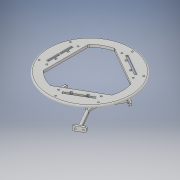
# Autodesk Inventor part: Stewart-Platform-Base-Außenanordnung
Saved by Autodesk Inventor 2018.2 (Build 222227000, 227)
## iProperties
Created: 2018-02-17
Part Number: Stewart-Platform-Base-Außenanordnung
Material: Generisch
Document SubType Name: Modeling
Designer: JochenAlt
Density: 1 g/cm^3
Appearance: Vorgabe
Author: JochenAlt
Autodesk Inventor part; units mm, degrees
ref_plane "YZ Plane" through (0, 0, 0) normal (1, 0, 0) x (0, 1, 0)
ref_plane "XZ Plane" through (0, 0, 0) normal (0, 1, 0) x (-1, 0, 0)
sketch "Skizze1" plane through (0, 0, 0) normal (0, 0, 1) x (1, 0, 0)
  line L0 (0, 96.3661) -> (0, -97.9027) construction
  line L1 (-96.2838, 0) -> (97.409, 0) construction
  line L2 (-57.6011, 28.85) -> (-45.1011, 28.85) construction
  line L3 (-41.8011, 25.55) -> (-41.8011, -25.55) construction
  line L4 (-45.1011, -28.85) -> (-57.6011, -28.85) construction
  line L5 (-60.9011, -25.55) -> (-60.9011, 25.55) construction
  arc A0 (-57.6011, 28.85) -> (-60.9011, 25.55) centre (-57.6011, 25.55) ccw construction
  arc A1 (-41.8011, 25.55) -> (-45.1011, 28.85) centre (-45.1011, 25.55) ccw construction
  arc A2 (-45.1011, -28.85) -> (-41.8011, -25.55) centre (-45.1011, -25.55) ccw construction
  arc A3 (-60.9011, -25.55) -> (-57.6011, -28.85) centre (-57.6011, -25.55) ccw construction
  circle A4 centre (-57.6011, 25.55) radius 1.3
  circle A5 centre (-45.1011, 25.55) radius 1.3
  circle A6 centre (-57.6011, -25.55) radius 1.3
  circle A7 centre (-45.1011, -25.55) radius 1.3
  line L6 (-47.8011, 20.25) -> (-47.8011, -20.25)
  line L7 (-50.9011, 20.25) -> (-50.9011, -20.25)
  line L8 (-50.9011, 20.25) -> (-47.8011, 20.25)
  line L9 (-50.9011, -20.25) -> (-47.8011, -20.25)
  line L10 (-50.9011, 0.8) -> (-47.8011, 0.8)
  line L11 (-50.9011, -0.8) -> (-47.8011, -0.8)
  line L12 (-47.8011, 11.55) -> (-44.7851, 11.55)
  line L13 (-44.7851, 11.55) -> (-44.7851, 8.75)
  line L14 (-44.7851, 8.75) -> (-47.8011, 8.75)
  line L15 (-47.8011, -8.75) -> (-44.7851, -8.75)
  line L16 (-44.7851, -8.75) -> (-44.7851, -11.55)
  line L17 (-44.7851, -11.55) -> (-47.8011, -11.55)
  line L18 (-45.1011, 29.15) -> (-57.6011, 29.15)
  arc A8 (-57.6011, 29.15) -> (-61.2011, 25.55) centre (-57.6011, 25.55) ccw
  line L19 (-61.2011, 25.55) -> (-61.2011, -25.55)
  arc A9 (-61.2011, -25.55) -> (-57.6011, -29.15) centre (-57.6011, -25.55) ccw
  line L20 (-57.6011, -29.15) -> (-45.1011, -29.15)
  arc A10 (-45.1011, -29.15) -> (-41.5011, -25.55) centre (-45.1011, -25.55) ccw
  line L21 (-41.5011, -25.55) -> (-41.5011, 25.55)
  arc A11 (-41.5011, 25.55) -> (-45.1011, 29.15) centre (-45.1011, 25.55) ccw
  line L22 (-63.3321, -28.8235) -> (-60.7271, -27.3356) construction
  line L23 (-39.5011, 0) -> (-41.5011, 0) construction
  circle A12 centre (0, 0) radius 39.5011 construction
  circle A13 centre (0, 0) radius 68.6134
  line L24 (-62.7201, 27.8206) -> (-60.8919, 27.0097) construction
  line L25 (-44.7851, -10.15) -> (-5.8601, -10.15) construction
  line L26 (6.3855, -31.3601) -> (-5.8601, -10.15) construction
  line L27 (-40.5011, -10.15) -> (-40.5011, -70.15) construction
  line L28 (11.4604, -40.15) -> (-40.5011, -70.15) construction
  line L29 (-41.5011, -19.95) -> (-47.8011, -19.95)
  line L30 (-41.5011, 19.95) -> (-47.8011, 19.95)
  arc A14 (47.7952, -24.4837) -> (42.8775, -23.166) centre (44.6775, -26.2837) ccw
  circle A15 centre (44.6775, -26.2837) radius 1.3
  line L31 (42.8775, -23.166) -> (-1.3764, -48.716)
  line L32 (38.0278, -25.966) -> (41.1778, -31.422)
  line L33 (32.3952, -33.0101) -> (33.9032, -35.622)
  line L34 (29.9703, -34.4101) -> (32.3952, -33.0101)
  line L35 (31.4783, -37.022) -> (29.9703, -34.4101)
  line L36 (6.3635, -51.522) -> (41.4376, -31.272)
  line L37 (42.9876, -33.9567) -> (41.4376, -31.272)
  line L38 (7.9135, -54.2067) -> (42.9876, -33.9567)
  line L39 (26.1434, -43.6817) -> (24.5934, -40.997)
  line L40 (24.7577, -44.4817) -> (23.2077, -41.797)
  line L41 (12.39, -44.5601) -> (14.8148, -43.1601)
  line L42 (14.8148, -43.1601) -> (16.3228, -45.772)
  line L43 (13.898, -47.172) -> (12.39, -44.5601)
  line L44 (3.4734, -45.916) -> (6.6234, -51.372)
  line L45 (7.9135, -54.2067) -> (6.3635, -51.522)
  arc A16 (-1.3764, -48.716) -> (-2.6941, -53.6337) centre (0.4236, -51.8337) ccw
  circle A17 centre (0.4236, -51.8337) radius 1.3
  line L46 (-2.6941, -53.6337) -> (3.5559, -64.459)
  circle A18 centre (50.9275, -37.109) radius 1.3
  arc A19 (52.7275, -40.2267) -> (54.0452, -35.309) centre (50.9275, -37.109) ccw
  line L47 (8.4736, -65.7767) -> (52.7275, -40.2267)
  circle A20 centre (6.6736, -62.659) radius 1.3
  arc A21 (3.5559, -64.459) -> (8.4736, -65.7767) centre (6.6736, -62.659) ccw
  line L48 (54.0452, -35.309) -> (47.7952, -24.4837)
  arc A22 (-2.6941, 53.6337) -> (-1.3764, 48.716) centre (0.4236, 51.8337) ccw
  circle A23 centre (0.4236, 51.8337) radius 1.3
  line L49 (-1.3764, 48.716) -> (42.8775, 23.166)
  line L50 (3.4734, 45.916) -> (6.6234, 51.372)
  line L51 (12.39, 44.5601) -> (13.898, 47.172)
  line L52 (14.8148, 43.1601) -> (12.39, 44.5601)
  line L53 (16.3228, 45.772) -> (14.8148, 43.1601)
  line L54 (41.4376, 31.272) -> (6.3635, 51.522)
  line L55 (7.9135, 54.2067) -> (6.3635, 51.522)
  line L56 (42.9876, 33.9567) -> (7.9135, 54.2067)
  line L57 (24.7577, 44.4817) -> (23.2077, 41.797)
  line L58 (26.1434, 43.6817) -> (24.5934, 40.997)
  line L59 (32.3952, 33.0101) -> (29.9703, 34.4101)
  line L60 (29.9703, 34.4101) -> (31.4783, 37.022)
  line L61 (33.9032, 35.622) -> (32.3952, 33.0101)
  line L62 (38.0278, 25.966) -> (41.1778, 31.422)
  line L63 (42.9876, 33.9567) -> (41.4376, 31.272)
  arc A24 (42.8775, 23.166) -> (47.7952, 24.4837) centre (44.6775, 26.2837) ccw
  circle A25 centre (44.6775, 26.2837) radius 1.3
  line L64 (47.7952, 24.4837) -> (54.0452, 35.309)
  circle A26 centre (6.6736, 62.659) radius 1.3
  arc A27 (8.4736, 65.7767) -> (3.5559, 64.459) centre (6.6736, 62.659) ccw
  line L65 (52.7275, 40.2267) -> (8.4736, 65.7767)
  circle A28 centre (50.9275, 37.109) radius 1.3
  arc A29 (54.0452, 35.309) -> (52.7275, 40.2267) centre (50.9275, 37.109) ccw
  line L66 (3.5559, 64.459) -> (-2.6941, 53.6337)
  line L67 (-39.5011, 36.0231) -> (-39.5011, -36.0231)
  line L68 (50.9475, -16.1974) -> (-11.4464, -52.2205)
  arc A30 (-53.749, 29.15) -> (-53.9107, 28.85) centre (0, 0) ccw
  arc A31 (-38.9435, -37.4086) -> (-12.9251, -52.4304) centre (0, 0) ccw
  line L69 (68.3365, 6.1578) -> (69.7386, 5.3484)
  arc A32 (51.8686, -15.0217) -> (51.8686, 15.0217) centre (0, 0) ccw
  arc A33 (-12.9251, 52.4304) -> (-38.9435, 37.4086) centre (0, 0) ccw
  line L70 (-30.7811, 63.3834) -> (-28.8354, 62.2601)
  line L71 (-11.4464, 52.2205) -> (50.9475, 16.1974)
  arc A34 (-39.5011, -36.0231) -> (-38.9435, -37.4086) centre (-37.5011, -36.0231) ccw
  arc A35 (-12.9251, -52.4304) -> (-11.4464, -52.2205) centre (-12.4464, -50.4885) ccw
  arc A36 (50.9475, -16.1974) -> (51.8686, -15.0217) centre (49.9475, -14.4654) ccw
  arc A37 (51.8686, 15.0217) -> (50.9475, 16.1974) centre (49.9475, 14.4654) ccw
  arc A38 (-11.4464, 52.2205) -> (-12.9251, 52.4304) centre (-12.4464, 50.4885) ccw
  arc A39 (-38.9435, 37.4086) -> (-39.5011, 36.0231) centre (-37.5011, 36.0231) ccw
  point P0 (0, 2)
  point P1 (-41.5011, -21.4)
  point P2 (-41.5011, 21.4)
  point P3 (20.7506, -35.941)
  point P4 (39.2835, -25.241)
  point P5 (2.2176, -46.641)
  point P6 (31.1827, -33.7101)
  point P7 (54.0368, -38.9234)
  point P8 (7.0549, -66.2388)
  point P9 (20.7506, 35.941)
  point P10 (2.2176, 46.641)
  point P11 (39.2835, 25.241)
  point P12 (13.6024, 43.8601)
  point P13 (6.6903, 66.259)
  point P14 (53.837, 39.2291)
  point P15 (-39.5011, 36.8193)
  point P16 (-39.5011, -36.8193)
  point P17 (51.637, -15.7993)
  point P18 (-12.1359, -52.6186)
  point P19 (51.637, 15.7993)
  point P20 (-12.1359, 52.6186)
  dimension "d1" = 57.7
  dimension "d2" = 19.1
  dimension "d3" = 3.3
  dimension "d5" = 2.6
  dimension "d6" = 6
  dimension "d7" = 3.1
  dimension "d9" = 1.6
  dimension "d10" = 2.984
  dimension "d11" = 2.8
  dimension "d12" = 17.5
  dimension "d21" = 0.3
  dimension "d22" = 3
  dimension "d34" = 2
  dimension "d35" = 2
  dimension "d40" = 1
  dimension "d42" = 60
  dimension "d43" = 137.2269
  dimension "d105" = 360
  dimension "d107" = 40.5
  dimension "d108" = 0.3
  dimension "d109" = 1
  dimension "d110" = 54
  dimension "d111" = 2
  constraints: 134 end point, 67 point on circle, 39 centre point, 33 point on line, 20 tangent, 14 coincident, 13 equal radius, 11 horizontal, 8 parallel, 6 perpendicular, 4 vertical, 3 line through centre, 2 midpoint, 1 collinear, 1 horizontal alignment, 258 other
  measures "d1" distance between parallel lines of L4 L2
  measures "d2" distance between parallel lines of L3 L5
  measures "d3" radius of A0
  measures "d5" diameter of A4
  measures "d9" distance between parallel lines of L11 L10
  measures "d10" distance between parallel lines of L3 L13
  measures "d11" distance between parallel lines of L14 L12
  measures "d12" distance between parallel lines of L15 L14
  measures "d21" distance between parallel lines of L19 L5
  measures "d22" distance of L22.end L22.start
  measures "d34" distance of L23.start L23.end
  measures "d35" distance of L24.start L24.end
  measures "d40" distance between parallel lines of L21 L27
  measures "d42" distance from line of L25 L27.end
  measures "d43" diameter of A13
  measures "d107" distance between parallel lines of L8 L9
  measures "d108" distance between parallel lines of L29 L9
  measures "d109" distance between parallel lines of L28 L31
  measures "d110" radius of A33
  measures "d111" radius of A34
extrude "Extrusion5" add sketch "Skizze1" along normal blind 4 contours L8 L7 L9 L6 L29 L21 A10 L20 A9 L19 A8 L18 A11 L30 | L30 L21 L29 L6 L17 L16 L15 L14 L13 L12 | L10 L6 L11 L7 | A13 | L48 A19 L47 A21 L46 A16 L31 L44 L36 L45 L38 L37 L32 A14 | L32 L36 L33 L34 L35 L42 L41 L43 L44 L31 | L66 A27 L65 A29 L64 A24 L49 L62 L54 L63 L56 L55 L50 A22 | L50 L54 L51 L52 L53 L60 L59 L61 L62 L49
extrude "Extrusion4" cut sketch "Skizze1" along normal blind 2 contours L8 L7 L9 L6 L29 L21 A10 L20 A9 L19 A8 L18 A11 L30 | L48 A19 L47 A21 L46 A16 L31 L44 L36 L45 L38 L37 L32 A14 | L66 A27 L65 A29 L64 A24 L49 L62 L54 L63 L56 L55 L50 A22
ref_plane "Arbeitsebene2" through (0, 0, -41.8) normal (0, 0, 1) x (1, 0, 0)
sketch "Skizze6" plane through (0, 0, -41.8) normal (0, 0, 1) x (1, 0, 0)
  line L0 (-47.8011, -0.8) -> (-47.8011, -8.75) construction
  line L1 (-47.8011, -8.75) -> (-44.7851, -8.75) construction
  line L2 (-44.7851, -8.75) -> (-44.7851, -11.55) construction
  line L3 (-44.7851, -11.55) -> (-47.8011, -11.55) construction
  line L4 (-47.8011, -11.55) -> (-47.8011, -20.25) construction
  line L5 (-47.8011, -20.25) -> (-50.9011, -20.25) construction
  line L6 (-50.9011, -20.25) -> (-50.9011, -0.8) construction
  line L7 (-47.8011, 20.25) -> (-47.8011, 11.55) construction
  line L8 (-47.8011, 11.55) -> (-44.7851, 11.55) construction
  line L9 (-44.7851, 11.55) -> (-44.7851, 8.75) construction
  line L10 (-44.7851, 8.75) -> (-47.8011, 8.75) construction
  line L11 (-50.9011, 20.25) -> (-47.8011, 20.25) construction
  circle A0 centre (-45.1011, -25.55) radius 1.3 construction
  circle A1 centre (-57.6011, -25.55) radius 1.3 construction
  circle A2 centre (-45.1011, 25.55) radius 1.3 construction
  circle A3 centre (-57.6011, 25.55) radius 1.3 construction
  circle A4 centre (0, 0) radius 68.6134 construction
  line L12 (-47.8011, -8.75) -> (-47.8011, 8.75)
  line L13 (-47.8011, -8.75) -> (-44.7851, -8.75)
  line L14 (-47.8011, 8.75) -> (-47.8011, -8.75) projected
  line L15 (-94.5835, 0) -> (94.5835, 0) construction
  line L16 (0, 94.5835) -> (0, -94.5835) construction
  line L17 (-44.7851, 8.75) -> (-44.7851, 2)
  line L18 (-44.7851, -2) -> (-44.7851, -8.75)
  line L19 (0, 0) -> (-8.9019, -15.4186) construction
  line L20 (0, 0) -> (-9.1171, 15.7912) construction
  arc A5 (-2.7017, -4.6795) -> (-12.7017, -2) centre (-12.7017, -22) ccw
  arc A6 (-12.7017, 2) -> (-2.7017, 4.6795) centre (-12.7017, 22) ccw
  line L21 (-2.7017, -4.6795) -> (0, -6.2393)
  line L22 (-2.7017, 4.6795) -> (0, 6.2393)
  line L23 (-44.7851, -2) -> (-12.7017, -2)
  line L24 (-44.7851, 2) -> (-12.7017, 2)
  line L25 (-44.7851, 8.75) -> (-47.8011, 8.75) projected
  line L26 (-47.8011, 8.75) -> (-44.7851, 8.75)
  arc A7 (0, 1.65) -> (0, -1.65) centre (0, 0) ccw
  line L27 (0, -6.2393) -> (0, -1.65)
  line L28 (0, 1.65) -> (0, 6.2393)
  line L29 (-47.8011, 8.75) -> (-47.8011, 0.8) projected
  line L30 (-47.8011, 0.8) -> (-50.9011, 0.8) projected
  line L31 (-50.9011, 0.8) -> (-50.9011, 20.25) projected
  line L32 (-50.9011, -0.8) -> (-47.8011, -0.8) projected
  dimension "d73" = 120
  dimension "d89" = 20
  dimension "d90" = 4
  dimension "d91" = 3.3
  constraints: 26 end point, 6 point on circle, 6 point on line, 5 perpendicular, 4 tangent, 3 centre point, 2 parallel, 1 coincident, 1 collinear, 1 symmetric about line, 1 vertical, 2 other
  measures "d73" angle of L20 L19
  measures "d89" radius of A6
  measures "d90" distance between parallel lines of L23 L24
  measures "d91" diameter of A7
extrude "Extrusion9" add sketch "Skizze6" against normal blind 7.1 separate body
sketch "Skizze7" plane through (-47.8011, -8.75, -41.8) normal (-1, 0, 0) x (0, 0, -1)
  circle A0 centre (3.8, -3.7) radius 1.3
  circle A1 centre (3.8, -13.8) radius 1.3
  line L0 (0, -17.5) -> (0, 0) construction
  line L1 (0, -8.75) -> (7.1, -8.75) construction
  line L2 (7.1, 0) -> (7.1, -17.5) construction
  point P0 (-41.8, -8.75)
  dimension "d76" = 2.6
  dimension "d77" = 10.1
  dimension "d88" = 3.3
  constraints: 2 centre point, 2 end point, 2 midpoint, 1 equal radius, 1 symmetric about line
  measures "d76" diameter of A1
  measures "d77" distance of A0.centre A1.centre
  measures "d88" distance from line of A0.centre L2
extrude "Extrusion10" cut sketch "Skizze7" against normal blind 10 bodies 1 2
pattern_circular "Runde Anordnung5" count 3 over 360 about axis through (0, 0, -10) along (0, 0, 1) of "Extrusion10", "Extrusion9" bodies 2
fillet "Rundung1" radius 2 30 edges at (-2.7017, -4.6795, -41.8) (-28.7434, -2, -41.8) (12.6397, -25.8925, -41.8) (-2.7017, 4.6795, -41.8) (12.6397, 25.8925, -41.8) (-28.7434, 2, -41.8) (16.1038, 23.8925, -41.8) (16.1038, -23.8925, -41.8) (5.4034, 0, -41.8) (-2.7017, -4.6795, -48.9) (-28.7434, -2, -48.9) (12.6397, -25.8925, -48.9) (16.1038, -23.8925, -48.9) (16.1038, 23.8925, -48.9) (5.4034, 0, -48.9) (-46.2931, 8.75, -48.9) (-46.2931, -8.75, -48.9) (15.5688, 44.466, -48.9) (30.7243, 35.716, -48.9) (30.7243, 35.716, -41.8) (15.5688, 44.466, -41.8) (-46.2931, 8.75, -41.8) (-46.2931, -8.75, -41.8) (15.5688, -44.466, -41.8) (15.5688, -44.466, -48.9) (30.7243, -35.716, -41.8) (30.7243, -35.716, -48.9) (12.6397, 25.8925, -48.9) (-28.7434, 2, -48.9) (-2.7017, 4.6795, -48.9)
fillet "Rundung2" radius 2 2 edges at (-68.3365, -6.1578, 4) (-68.3365, -6.1578, 0)
equation "\"d22\" = d20"
equation "\"d35\" = d34"
equation "\"d44\" = d21"
equation "\"d20\" = 3"
